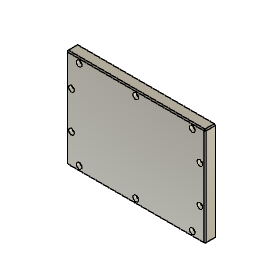
CAD_File 8 (Autodesk Fusion 360 design; units mm, degrees)
Autodesk Fusion 360 part; units mm, degrees
sketch "Sketch1" plane through (0, -115, 0) normal (0, -1, 0) x (1, 0, 0)
  line L0 (-115, -20) -> (-135, -20)
  line L1 (-135, -20) -> (-135, -172.35)
  line L2 (-135, -172.35) -> (-115, -172.35)
  line L3 (-115, -172.35) -> (-115, -20)
  line L4 (-135, -20) -> (-135, -172.35)
  line L5 (-135, 0) -> (-135, -20)
  line L6 (135, 0) -> (-135, 0)
  line L7 (135, 0) -> (135, -20)
  line L8 (135, -20) -> (135, -172.35)
  line L9 (135, -172.35) -> (135, -192.35)
  line L10 (135, -192.35) -> (-135, -192.35)
  line L11 (-135, -172.35) -> (-135, -192.35)
extrude "Extrude1" add sketch "Sketch1" along normal blind 20
chamfer "Chamfer1" distance 2 angle 45 8 edges at (-135, -135, -96.175) (0, -135, 0) (135, -135, -96.175) (0, -135, -192.35) (-135, -125, -192.35) (-135, -125, 0) (135, -125, 0) (135, -125, -192.35)
sketch "Sketch2" plane through (0, -135, 0) normal (0, -1, 0) x (1, 0, 0)
  line L0 (-133, -190.35) -> (133, -190.35)
  line L1 (133, -190.35) -> (133, -2)
  line L2 (133, -2) -> (-133, -2)
  line L3 (-133, -2) -> (-133, -190.35)
  circle A0 centre (110, -10) radius 3
  circle A1 centre (110, -10) radius 5.5
  circle A2 centre (125, -60) radius 3
  circle A3 centre (125, -60) radius 5.5
  circle A4 centre (0, -10) radius 3
  circle A5 centre (0, -10) radius 5.5
  circle A6 centre (-110, -10) radius 3
  circle A7 centre (-110, -10) radius 5.5
  circle A8 centre (-125, -60) radius 3
  circle A9 centre (-125, -60) radius 5.5
  circle A10 centre (-125, -132.35) radius 3
  circle A11 centre (-125, -132.35) radius 5.5
  circle A12 centre (-110, -182.35) radius 3
  circle A13 centre (-110, -182.35) radius 5.5
  circle A14 centre (0, -182.35) radius 3
  circle A15 centre (0, -182.35) radius 5.5
  circle A16 centre (110, -182.35) radius 3
  circle A17 centre (110, -182.35) radius 5.5
  circle A18 centre (125, -132.35) radius 3
  circle A19 centre (125, -132.35) radius 5.5
extrude "Extrude2" cut sketch "Sketch2" against normal blind 40 contours A0 | A2 | A4 | A6 | A8 | A10 | A12 | A14 | A16 | A18
extrude "Extrude3" cut sketch "Sketch2" against normal blind 6.5 contours A1 | A3 | A5 | A7 | A9 | A11 | A13 | A15 | A17 | A19
sketch "Sketch3" plane through (0, -115, 0) normal (0, 1, 0) x (-1, 0, 0)
  circle A0 centre (0, -182.35) radius 3
  circle A1 centre (-110, -10) radius 3
  circle A2 centre (125, -60) radius 3
  circle A3 centre (-125, -60) radius 3
  circle A4 centre (110, -182.35) radius 3
  circle A5 centre (-110, -182.35) radius 3
  circle A6 centre (0, -10) radius 3
  circle A7 centre (110, -10) radius 3
  circle A8 centre (-125, -132.35) radius 3
  circle A9 centre (125, -132.35) radius 3
  line L0 (-135, -190.35) -> (-133, -192.35)
  line L1 (-133, -192.35) -> (133, -192.35)
  line L2 (133, -192.35) -> (135, -190.35)
  line L3 (135, -190.35) -> (135, -2)
  line L4 (135, -2) -> (133, 0)
  line L5 (133, 0) -> (-133, 0)
  line L6 (-133, 0) -> (-135, -2)
  line L7 (-135, -2) -> (-135, -190.35)
  line L8 (2.9509, -155.0955) -> (1.7299, -155.191)
  spline S0 degree 2 poles (1.7299, -155.191) (1.5662, -154.4679) (1.266, -154.1405) knots 0 0 0 1 1 1
  spline S1 degree 2 poles (1.266, -154.1405) (0.7681, -153.6153) (0.0382, -153.6153) knots 0 0 0 1 1 1
  spline S2 degree 2 poles (0.0382, -153.6153) (-0.5484, -153.6153) (-0.9918, -153.9427) knots 0 0 0 1 1 1
  spline S3 degree 2 poles (-0.9918, -153.9427) (-1.5716, -154.3656) (-1.9059, -155.1774) knots 0 0 0 1 1 1
  spline S4 degree 2 poles (-1.9059, -155.1774) (-2.2401, -155.9891) (-2.2538, -157.4898) knots 0 0 0 1 1 1
  spline S5 degree 2 poles (-2.2538, -157.4898) (-1.8104, -156.8145) (-1.1692, -156.487) knots 0 0 0 1 1 1
  spline S6 degree 2 poles (-1.1692, -156.487) (-0.528, -156.1596) (0.1746, -156.1596) knots 0 0 0 1 1 1
  spline S7 degree 2 poles (0.1746, -156.1596) (1.4025, -156.1596) (2.2653, -157.0634) knots 0 0 0 1 1 1
  spline S8 degree 2 poles (2.2653, -157.0634) (3.1282, -157.9673) (3.1282, -159.3997) knots 0 0 0 1 1 1
  spline S9 degree 2 poles (3.1282, -159.3997) (3.1282, -160.3411) (2.7224, -161.1494) knots 0 0 0 1 1 1
  spline S10 degree 2 poles (2.7224, -161.1494) (2.3165, -161.9577) (1.6071, -162.3875) knots 0 0 0 1 1 1
  spline S11 degree 2 poles (1.6071, -162.3875) (0.8977, -162.8172) (-0.0027, -162.8172) knots 0 0 0 1 1 1
  spline S12 degree 2 poles (-0.0027, -162.8172) (-1.5375, -162.8172) (-2.5061, -161.6883) knots 0 0 0 1 1 1
  spline S13 degree 2 poles (-2.5061, -161.6883) (-3.4748, -160.5593) (-3.4748, -157.9673) knots 0 0 0 1 1 1
  spline S14 degree 2 poles (-3.4748, -157.9673) (-3.4748, -155.0682) (-2.4038, -153.7517) knots 0 0 0 1 1 1
  spline S15 degree 2 poles (-2.4038, -153.7517) (-1.4693, -152.6057) (0.1132, -152.6057) knots 0 0 0 1 1 1
  spline S16 degree 2 poles (0.1132, -152.6057) (1.2933, -152.6057) (2.0471, -153.2674) knots 0 0 0 1 1 1
  spline S17 degree 2 poles (2.0471, -153.2674) (2.8008, -153.9291) (2.9509, -155.0955) knots 0 0 0 1 1 1
  spline S18 degree 2 poles (-2.0628, -159.4066) (-2.0628, -160.0409) (-1.7933, -160.6207) knots 0 0 0 1 1 1
  spline S19 degree 2 poles (-1.7933, -160.6207) (-1.5239, -161.2005) (-1.0396, -161.5041) knots 0 0 0 1 1 1
  spline S20 degree 2 poles (-1.0396, -161.5041) (-0.5553, -161.8076) (-0.0232, -161.8076) knots 0 0 0 1 1 1
  spline S21 degree 2 poles (-0.0232, -161.8076) (0.7544, -161.8076) (1.3138, -161.1801) knots 0 0 0 1 1 1
  spline S22 degree 2 poles (1.3138, -161.1801) (1.8731, -160.5525) (1.8731, -159.4748) knots 0 0 0 1 1 1
  spline S23 degree 2 poles (1.8731, -159.4748) (1.8731, -158.4379) (1.3206, -157.8411) knots 0 0 0 1 1 1
  spline S24 degree 2 poles (1.3206, -157.8411) (0.7681, -157.2442) (-0.0709, -157.2442) knots 0 0 0 1 1 1
  spline S25 degree 2 poles (-0.0709, -157.2442) (-0.9031, -157.2442) (-1.4829, -157.8411) knots 0 0 0 1 1 1
  spline S26 degree 2 poles (-1.4829, -157.8411) (-2.0628, -158.4379) (-2.0628, -159.4066) knots 0 0 0 1 1 1
extrude "Extrude4" cut sketch "Sketch3" against normal blind 0.2 contours L8 S0 S1 S2 S3 S4 S5 S6 S7 S8 S9 S10 S11 S12 S13 S14 S15 S16 S17
